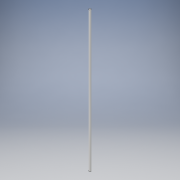
# Autodesk Inventor part: Barre Circulaire
Saved by Autodesk Inventor 2019 (Build 230136000, 136)
## iProperties
Created: 2020-03-11
Part Number: Barre Circulaire
Material: Générique
Document SubType Name: Modeling
Designer: Quentin
Density: 1 g/cm^3
Appearance: Par défaut
Author: Quentin
Autodesk Inventor part; units mm, degrees
ref_plane "YZ Plane" through (0, 0, 0) normal (1, 0, 0) x (0, 1, 0)
ref_plane "XZ Plane" through (0, 0, 0) normal (0, 1, 0) x (-1, 0, 0)
ref_plane "XY Plane" through (0, 0, 0) normal (0, 0, 1) x (1, 0, 0)
sketch "Esquisse1" plane through (0, 0, 0) normal (0, 0, 1) x (1, 0, 0)
  line L0 (0, 0) -> (0, 140.38)
  line L1 (0, 140.38) -> (1, 140.38)
  line L2 (1, 140.38) -> (1, 0)
  line L3 (1, 0) -> (0, 0)
  dimension "d0" = 140.38
  dimension "d1" = 1
  constraints: 8 end point, 2 perpendicular, 1 parallel, 1 vertical
  measures "d0" distance of L0.start L0.end
  measures "d1" distance of L0.end L1.end
revolve "Révolution1" add sketch "Esquisse1" angle 360 about axis through (1, 140.38, 0) along (0, -1, 0)
